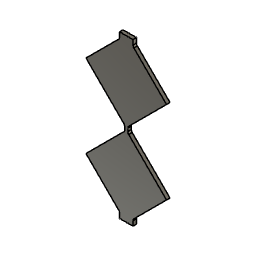
Hourglass Backcover (Autodesk Fusion 360 design; units mm, degrees)
Autodesk Fusion 360 part; units mm, degrees
sketch "back" plane through (0, 0, 0) normal (0, 1, 0) x (1, 0, 0)
  arc A0 (-49, 26.4274) -> (-48.5607, 25.3667) centre (-47.5, 26.4274) ccw
  line L0 (-46, -19.363) -> (-54, -19.363)
  line L1 (-54.4393, -15.4237) -> (-73.3345, 3.4715)
  arc A1 (-48.5607, 29.2454) -> (-49, 28.1847) centre (-47.5, 28.1847) ccw
  line L2 (-48.5607, 25.3667) -> (-26.6655, 3.4715)
  arc A2 (-54, -16.4843) -> (-54.4393, -15.4237) centre (-55.5, -16.4843) ccw
  arc A3 (-51.4393, 25.3667) -> (-51, 26.4274) centre (-52.5, 26.4274) ccw
  arc A4 (-54.4393, 70.0358) -> (-54, 71.0964) centre (-55.5, 71.0964) ccw
  line L3 (-73.1931, 51.1406) -> (-54.3686, 69.965)
  arc A5 (-54.3686, 69.965) -> (-53.9, 71.0964) centre (-55.5, 71.0964) ccw
  line L4 (-53.9, -19.263) -> (-53.9, -16.4843)
  line L5 (-45.5607, 70.0358) -> (-26.6655, 51.1406)
  line L6 (-51, 26.4274) -> (-51, 28.1847)
  line L7 (-46.1, 73.8751) -> (-46.1, 71.0964)
  line L8 (-46.1, -16.4843) -> (-46.1, -19.263)
  arc A6 (-46, 71.0964) -> (-45.5607, 70.0358) centre (-44.5, 71.0964) ccw
  arc A7 (-45.5607, -15.4237) -> (-46, -16.4843) centre (-44.5, -16.4843) ccw
  line L9 (-54, 71.0964) -> (-54, 73.9751)
  arc A8 (-51, 28.1847) -> (-51.4393, 29.2454) centre (-52.5, 28.1847) ccw
  line L10 (-46, 73.9751) -> (-46, 71.0964)
  line L11 (-26.6655, 3.4715) -> (-45.5607, -15.4237)
  line L12 (-45.6314, 69.965) -> (-26.8069, 51.1406)
  arc A9 (-50.9, 28.1847) -> (-51.3686, 29.3161) centre (-52.5, 28.1847) ccw
  line L13 (-46, -16.4843) -> (-46, -19.363)
  line L14 (-54, -19.363) -> (-54, -16.4843)
  line L15 (-54, 73.9751) -> (-46, 73.9751)
  line L16 (-26.6655, 51.1406) -> (-48.5607, 29.2454)
  line L17 (-51.4393, 29.2454) -> (-73.3345, 51.1406)
  line L18 (-54.3686, -15.353) -> (-73.1931, 3.4715)
  arc A10 (-48.6314, 29.3161) -> (-49.1, 28.1847) centre (-47.5, 28.1847) ccw
  line L19 (-73.3345, 3.4715) -> (-51.4393, 25.3667)
  arc A11 (-51.3686, 25.296) -> (-50.9, 26.4274) centre (-52.5, 26.4274) ccw
  arc A12 (-49.1, 26.4274) -> (-48.6314, 25.296) centre (-47.5, 26.4274) ccw
  line L20 (-50.9, 26.4274) -> (-50.9, 28.1847)
  line L21 (-73.3345, 51.1406) -> (-54.4393, 70.0358)
  line L22 (-53.9, 71.0964) -> (-53.9, 73.8751)
  line L23 (-49, 28.1847) -> (-49, 26.4274)
  arc A13 (-46.1, 71.0964) -> (-45.6314, 69.965) centre (-44.5, 71.0964) ccw
  line L24 (-49.1, 28.1847) -> (-49.1, 26.4274)
  arc A14 (-45.6314, -15.353) -> (-46.1, -16.4843) centre (-44.5, -16.4843) ccw
  line L25 (-26.8069, 3.4715) -> (-45.6314, -15.353)
  arc A15 (-53.9, -16.4843) -> (-54.3686, -15.353) centre (-55.5, -16.4843) ccw
  line L26 (-26.8069, 51.1406) -> (-48.6314, 29.3161)
  line L27 (-73.1931, 3.4715) -> (-51.3686, 25.296)
  line L28 (-51.3686, 29.3161) -> (-73.1931, 51.1406)
  line L29 (-48.6314, 25.296) -> (-26.8069, 3.4715)
  line L30 (-46.1, -19.263) -> (-53.9, -19.263)
  line L31 (-53.9, 73.8751) -> (-46.1, 73.8751)
extrude "Extrude1" add sketch "back" along normal blind 2 contours L3 A5 L4 L7 L8 L12 A9 L18 A10 A11 A12 L20 L22 A13 L24 A14 L25 A15 L26 L27 L28 L29 L30 L31
